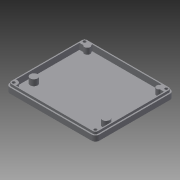
# Autodesk Inventor part: pablogilLCDCaseBottom
Saved by Autodesk Inventor 2015 SP1 (Build 190203100, 203)
## iProperties
Created: 2015-04-16
Part Number: pablogilLCDCaseBottom
Material: Generic
Document SubType Name: Modeling
Designer: Jack
Density: 1 g/cm^3
Appearance: Default
Author: Jack
Autodesk Inventor part; units mm, degrees
ref_plane "YZ Plane" through (0, 0, 0) normal (1, 0, 0) x (0, 1, 0)
ref_plane "XZ Plane" through (0, 0, 0) normal (0, 1, 0) x (-1, 0, 0)
ref_plane "XY Plane" through (0, 0, 0) normal (0, 0, 1) x (1, 0, 0)
sketch "Sketch1" plane through (0, 0, 0) normal (0, 0, 1) x (1, 0, 0)
  line L0 (0, 0) -> (-108.6, 0)
  line L1 (-108.6, 0) -> (-108.6, 95.4)
  line L2 (-108.6, 95.4) -> (0, 95.4)
  line L3 (0, 95.4) -> (0, 0)
  dimension "d0" = 108.6
  dimension "d1" = 95.4
  constraints: 8 end point, 2 parallel, 1 horizontal, 1 perpendicular
  measures "d0" distance of L1.end L2.end
  measures "d1" distance of L0.end L1.end
extrude "Extrusion1" add sketch "Sketch1" along normal blind 2
sketch "Sketch2" plane through (0, 0, 2) normal (0, 0, 1) x (1, 0, 0)
  line L0 (-108.6, 0) -> (0, 0) projected
  line L1 (0, 0) -> (0, 95.4) projected
  line L2 (0, 95.4) -> (-108.6, 95.4) projected
  line L3 (-108.6, 95.4) -> (-108.6, 0) projected
  line L4 (-107, 93.8) -> (-1.6, 93.8)
  line L5 (-1.6, 93.8) -> (-1.6, 1.6)
  line L6 (-1.6, 1.6) -> (-107, 1.6)
  line L7 (-107, 1.6) -> (-107, 93.8)
  dimension "d4" = 1.6
  constraints: 8 end point, 3 other
  measures "d4" distance between parallel lines of L2 L4
extrude "Extrusion2" add sketch "Sketch2" along normal blind 4.5
sketch "Sketch3" plane through (0, 0, 2) normal (0, 0, 1) x (1, 0, 0)
  line L0 (-1.6, 1.6) -> (-1.6, 93.8) projected
  line L1 (-1.6, 93.8) -> (-107, 93.8) projected
  line L2 (-107, 93.8) -> (-107, 1.6) projected
  line L3 (-107, 1.6) -> (-1.6, 1.6) projected
  line L4 (-105.6, 92.4) -> (-3, 92.4)
  line L5 (-3, 92.4) -> (-3, 3)
  line L6 (-3, 3) -> (-105.6, 3)
  line L7 (-105.6, 3) -> (-105.6, 92.4)
  point P0 (0, 0)
  dimension "d7" = 1.4
  constraints: 8 end point, 3 other
  measures "d7" distance between parallel lines of L1 L4
extrude "Extrusion3" add sketch "Sketch3" along normal blind 7.3
sketch "Sketch4" plane through (0, 0, 2) normal (0, 0, 1) x (1, 0, 0)
  line L0 (-3, 3) -> (-3, 92.4) projected
  line L1 (-105.6, 92.4) -> (-105.6, 3) projected
  line L2 (-105.6, 3) -> (-3, 3) projected
  circle A0 centre (-98.1, 23.4) radius 4.5
  circle A1 centre (-10.5, 23.4) radius 4.5
  point P0 (0, 0)
  dimension "d10" = 9
  dimension "d11" = 20.4
  dimension "d12" = 7.5
  dimension "d13" = 7.5
  constraints: 2 centre point, 1 equal radius, 1 horizontal alignment
  measures "d10" diameter of A0
  measures "d11" distance from line of L2 A0.centre
  measures "d12" distance from line of L0 A1.centre
  measures "d13" distance from line of L1 A0.centre
extrude "Extrusion4" add sketch "Sketch4" along normal blind 7.3
sketch "Sketch5" plane through (0, 0, 9.3) normal (0, 0, 1) x (1, 0, 0)
  line L0 (-3, 92.4) -> (-3, 3) projected
  line L1 (-3, 3) -> (-105.6, 3) projected
  line L2 (-105.6, 3) -> (-105.6, 92.4) projected
  line L3 (-105.6, 92.4) -> (-3, 92.4) projected
  line L4 (-105.6, 92.4) -> (-105.6, 3) projected
  line L5 (-3, 92.4) -> (-105.6, 92.4) projected
  line L6 (-105.6, 3) -> (-3, 3) projected
  arc A0 (-4.7, 9.2) -> (-9.2, 4.7) centre (-4.7, 4.7) ccw
  line L7 (-3, 3) -> (-3, 92.4) projected
  line L8 (-4.7, 9.2) -> (-3, 9.2)
  line L9 (-9.2, 4.7) -> (-9.2, 3)
  line L10 (-103.9, 9.2) -> (-105.6, 9.2)
  line L11 (-99.4, 4.7) -> (-99.4, 3)
  arc A1 (-99.4, 4.7) -> (-103.9, 9.2) centre (-103.9, 4.7) ccw
  arc A2 (-100.9723, 86.2) -> (-96.2, 91.1394) centre (-98.1, 88.2) ccw
  arc A3 (-12.4, 91.1394) -> (-7.6277, 86.2) centre (-10.5, 88.2) ccw
  line L12 (-105.6, 86.2) -> (-100.9723, 86.2)
  line L13 (-96.2, 91.1394) -> (-96.2, 92.4)
  line L14 (-12.4, 91.1394) -> (-12.4, 92.4)
  line L15 (-7.6277, 86.2) -> (-3, 86.2)
  point P0 (0, 0)
  point P1 (-103.9, 90.7)
  point P2 (-4.7, 90.7)
  dimension "d16" = 1.7
  dimension "d17" = 1.7
  dimension "d18" = 1.7
  dimension "d19" = 1.7
  dimension "d21" = 4.5
  dimension "d22" = 7.5
  dimension "d23" = 4.2
  dimension "d24" = 7.5
  dimension "d25" = 4.2
  dimension "d26" = 7
  dimension "d27" = 6.2
  dimension "d28" = 9.4
  constraints: 16 end point, 10 point on line, 8 point on circle, 6 perpendicular, 4 centre point, 4 coincident, 3 horizontal alignment, 3 tangent, 2 equal length, 2 equal radius, 2 vertical alignment
  measures "d16" distance from line of L0 point (-4.7, 4.7)
  measures "d17" distance from line of L1 point (-4.7, 4.7)
  measures "d18" distance from line of L2 point (-103.9, 4.7)
  measures "d19" distance from line of L3 point (-103.9, 90.7)
  measures "d21" radius of A0
  measures "d22" distance from line of L2 point (-98.1, 88.2)
  measures "d23" distance from line of L3 point (-98.1, 88.2)
  measures "d24" distance from line of L0 point (-10.5, 88.2)
  measures "d25" distance from line of L3 point (-10.5, 88.2)
  measures "d26" diameter of A2
  measures "d27" distance between parallel lines of L3 L12
  measures "d28" distance between parallel lines of L2 L13
extrude "Extrusion5" add sketch "Sketch5" against normal up to next contours L0 L15 A3 L14 L3 | L0 L1 L9 A0 L8 | L13 A2 L12 L2 L3 | L1 L2 L10 A1 L11
fillet "Fillet1" radius 4.7 4 edges at (-108.6, 0, 3.25) (0, 0, 3.25) (0, 95.4, 3.25) (-108.6, 95.4, 3.25)
fillet "Fillet2" radius 3.1 4 edges at (-107, 93.8, 7.9) (-107, 1.6, 7.9) (-1.6, 1.6, 7.9) (-1.6, 93.8, 7.9)
sketch "Sketch6" plane through (0, 0, 0) normal (0, 0, -1) x (-1, 0, 0)
  arc A0 (108.6, 90.7) -> (103.9, 95.4) centre (103.9, 90.7) ccw projected
  arc A1 (4.7, 95.4) -> (0, 90.7) centre (4.7, 90.7) ccw projected
  arc A2 (0, 4.7) -> (4.7, 0) centre (4.7, 4.7) ccw projected
  arc A3 (103.9, 0) -> (108.6, 4.7) centre (103.9, 4.7) ccw projected
  point P0 (0, 0)
hole "Hole1" at (-4.7, 90.7, 0) at (-103.9, 90.7, 0) at (-4.7, 4.7, 0) at (-103.9, 4.7, 0) direction (0, 0, 1) diameter 3.5 end up to face face through (-40.3333, 93.3333, 9.3) facing (0, 0, 1) counterbore diameter 5.8 counterbore depth 6
body "Solid1"
